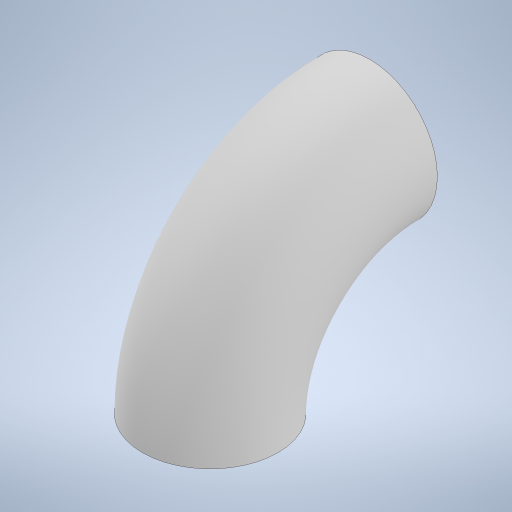
# Autodesk Inventor part: 05-22-2023 curva Sweep
Saved by Autodesk Inventor 2023 (Build 270158000, 158)
## iProperties
Created: 2023-05-22
Part Number: 05-22-2023 curva Sweep
Material: Generico
Document SubType Name: Modeling
Designer: Admin
Density: 1 g/cm^3
Appearance: Default
Author: Admin
Autodesk Inventor part; units mm, degrees
ref_plane "YZ Plane" through (0, 0, 0) normal (1, 0, 0) x (0, 1, 0)
ref_plane "XZ Plane" through (0, 0, 0) normal (0, 1, 0) x (-1, 0, 0)
ref_plane "XY Plane" through (0, 0, 0) normal (0, 0, 1) x (1, 0, 0)
sketch "Schizzo1" plane through (0, 0, 0) normal (0, 1, 0) x (-1, 0, 0)
  circle A0 centre (0, 0) radius 75
  circle A1 centre (0, 0) radius 85
  dimension "d0" = 150
  dimension "d1" = 170
  constraints: 2 centre point, 2 coincident
  measures "d0" diameter of A0
  measures "d1" diameter of A1
sketch "Schizzo2" plane through (0, 0, 0) normal (1, 0, 0) x (0, 1, 0)
  arc A0 (200, -200) -> (0, 0) centre (0, -200) ccw
  dimension "d2" = 200
  constraints: 2 point on circle, 1 centre point, 1 horizontal alignment, 1 vertical alignment
  measures "d2" radius of A0
sweep "Sweep1" add profiles "Schizzo1" path "Schizzo2"
